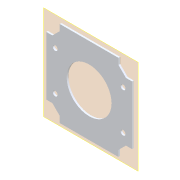
# Autodesk Inventor part: 20_Cube_Insert_XY_manipulator_lid_v3
Saved by Autodesk Inventor 2022 (Build 260153000, 153)
## iProperties
Created: 2021-12-16
Part Number: 20_Cube_Insert_XY_manipulator_lid_v3
Material: Generisch
Document SubType Name: Modeling
Designer: diederichbenedict
Density: 1 g/cm^3
Appearance: Vorgabe
Author: diederichbenedict
Autodesk Inventor part; units mm, degrees
ref_plane "YZ Plane" through (0, 0, 0) normal (1, 0, 0) x (0, 1, 0)
ref_plane "XZ Plane" through (0, 0, 0) normal (0, 1, 0) x (-1, 0, 0)
ref_plane "XY Plane" through (0, 0, 0) normal (0, 0, 1) x (1, 0, 0)
ref_plane "Arbeitsebene1" through (0, 0, 0) normal (0, 0, 1) x (1, 0, 0)
sketch "Skizze1" plane through (0, 0, 0) normal (0, 0, 1) x (1, 0, 0)
  circle A0 centre (-3.3862, 11.51) radius 1.4 projected
  circle A1 centre (-42.7562, -11.35) radius 1.4 projected
  circle A2 centre (-42.7562, 11.51) radius 1.4 projected
  circle A3 centre (-3.3862, -11.35) radius 1.4 projected
  circle A4 centre (-23.0712, 0.08) radius 13 projected
  line L0 (-6.1126, -24.9) -> (-40.0712, -24.9) projected
  line L1 (-40.0712, -24.9) -> (-40.0712, -21.3252) projected
  line L2 (-40.0712, -21.3252) -> (-44.3964, -17) projected
  line L3 (-44.3964, -17) -> (-47.9712, -17) projected
  line L4 (-47.9712, -17) -> (-47.9712, 17) projected
  line L5 (-47.9712, 17) -> (-44.3964, 17) projected
  line L6 (-44.3964, 17) -> (-40.0712, 21.3252) projected
  line L7 (-40.0712, 21.3252) -> (-40.0712, 24.9) projected
  line L8 (-40.0712, 24.9) -> (-6.0712, 24.9) projected
  line L9 (-6.0712, 24.9) -> (-6.0712, 21.3252) projected
  line L10 (-6.0712, 21.3252) -> (-1.746, 17) projected
  line L11 (-1.746, 17) -> (1.8288, 17) projected
  line L12 (1.8288, 17) -> (1.8288, -17) projected
  line L13 (1.8288, -17) -> (-1.746, -17) projected
  line L14 (-1.746, -17) -> (-6.1126, -21.3666) projected
  line L15 (-6.1126, -21.3666) -> (-6.1126, -24.9) projected
  point P0 (0, 0)
extrude "Extrusion1" add sketch "Skizze1" along normal blind 1
